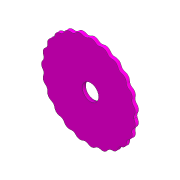
# Autodesk Inventor part: epicycloid
Saved by Autodesk Inventor 2022 (Build 260153000, 153)
## iProperties
Created: 2023-11-18
Part Number: epicycloid
Material: 一般
Document SubType Name: Modeling
Designer: JOU
Density: 1 g/cm^3
Appearance: 預設
Author: JOU
Autodesk Inventor part; units mm, degrees
ref_plane "YZ Plane" through (0, 0, 0) normal (1, 0, 0) x (0, 1, 0)
ref_plane "XZ Plane" through (0, 0, 0) normal (0, 1, 0) x (-1, 0, 0)
ref_plane "XY Plane" through (0, 0, 0) normal (0, 0, 1) x (1, 0, 0)
sketch "草圖1" plane through (0, 0, 0) normal (0, 0, 1) x (1, 0, 0)
  spline S0 degree 3 poles (138.6565, -4.115) (139.0078, -5.0402) (139.622, -6.6578) (140.7346, -8.8016) (141.6039, -10.7606) (142.2908, -12.8288) (142.7395, -15.1027) (142.8776, -17.5459) (142.6548, -20.0506) (142.0718, -22.4816) (141.1815, -24.7182) (140.0679, -26.6922) (138.8, -28.425) (137.3588, -30.0737) (135.6, -32.0105) (133.6246, -34.7946) (132.3649, -38.5247) (132.3554, -42.1634) (132.8434, -44.9603) (133.2666, -47.1894) (133.5136, -49.3089) (133.5257, -51.532) (133.2299, -53.8808) (132.5764, -56.2723) (131.5654, -58.5796) (130.2524, -60.6783) (128.7308, -62.4839) (127.0941, -63.9798) (125.3716, -65.2386) (123.4392, -66.4555) (121.0392, -68.0358) (118.3954, -70.5774) (116.5842, -74.0652) (115.9348, -77.381) (115.726, -79.9601) (115.4995, -82.13) (115.0882, -84.2405) (114.3916, -86.404) (113.3491, -88.5798) (111.9559, -90.6584) (110.2664, -92.519) (108.3804, -94.0712) (106.4106, -95.2802) (104.4306, -96.1793) (102.3977, -96.8704) (100.0593, -97.5478) (97.0906, -98.6367) (93.9043, -100.8025) (91.6334, -103.8672) (90.4103, -106.7035) (89.5885, -108.949) (88.7489, -110.9181) (87.693, -112.8302) (86.3231, -114.7076) (84.6177, -116.4688) (82.6244, -118.0035) (80.4443, -119.2217) (78.2018, -120.082) (76.0022, -120.6018) (73.8722, -120.8478) (71.6744, -120.9144) (69.029, -120.956) (65.6165, -121.4494) (62.0504, -123.1305) (59.4348, -125.6172) (57.7521, -127.8616) (56.4166, -129.6789) (55.0289, -131.3009) (53.3999, -132.8226) (51.4684, -134.2015) (49.2643, -135.3439) (46.8828, -136.1647) (44.4535, -136.6216) (42.1006, -136.7277) (39.897, -136.5414) (37.803, -136.1333) (35.5805, -135.5443) (32.7506, -134.8724) (29.059, -134.7182) (25.2982, -135.8285) (22.4771, -137.623) (20.4734, -139.2159) (18.7352, -140.5221) (16.9037, -141.6552) (14.8359, -142.614) (12.5248, -143.3247) (10.0501, -143.7098) (7.5383, -143.729) (5.1234, -143.3958) (2.9049, -142.7703) (0.9048, -141.9288) (-0.988, -140.9064) (-3.0992, -139.648) (-5.9637, -138.2247) (-9.7496, -137.4239) (-13.5121, -137.9045) (-16.3794, -138.9508) (-18.5632, -139.8737) (-20.5757, -140.5959) (-22.7016, -141.1198) (-25.0165, -141.3873) (-27.4717, -141.3277) (-29.9522, -140.9025) (-32.3231, -140.1264) (-34.4711, -139.0641) (-36.3401, -137.8045) (-37.9655, -136.4101) (-39.5172, -134.8386) (-41.3782, -132.9154) (-44.1155, -130.7638) (-47.8029, -129.3589) (-51.3772, -129.1863) (-54.132, -129.4936) (-56.3593, -129.7521) (-58.4935, -129.836) (-60.7226, -129.6717) (-63.0517, -129.1861) (-65.3888, -128.3392) (-67.6062, -127.1449) (-69.586, -125.6711) (-71.2554, -124.0184) (-72.6107, -122.2781) (-73.7347, -120.4643) (-74.8264, -118.422) (-76.2957, -115.8709) (-78.7548, -113.078) (-82.1531, -111.1423) (-85.3623, -110.3412) (-87.8678, -109.9704) (-90.0011, -109.5863) (-92.0802, -109.0105) (-94.1933, -108.1393) (-96.2872, -106.9199) (-98.2495, -105.3604) (-99.9652, -103.528) (-101.3549, -101.5309) (-102.3974, -99.4824) (-103.1361, -97.4468) (-103.6752, -95.3592) (-104.2022, -92.934) (-105.1501, -89.8407) (-107.2041, -86.5431) (-110.1376, -84.1744) (-112.8343, -82.8242) (-114.981, -81.8643) (-116.8771, -80.8802) (-118.7093, -79.6719) (-120.4808, -78.1482) (-122.1043, -76.2998) (-123.4736, -74.1873) (-124.5092, -71.9208) (-125.1834, -69.6272) (-125.5254, -67.4058) (-125.6061, -65.268) (-125.511, -63.0511) (-125.3803, -60.3469) (-125.7145, -56.8481) (-127.26, -53.2155) (-129.5824, -50.5344) (-131.6676, -48.7582) (-133.3645, -47.311) (-134.8771, -45.8009) (-136.2729, -44.0472) (-137.4984, -42.0012) (-138.4614, -39.7061) (-139.0864, -37.2668) (-139.3449, -34.8162) (-139.2628, -32.4748) (-138.9056, -30.3038) (-138.3389, -28.2455) (-137.5833, -26.0381) (-136.725, -23.1846) (-136.4072, -19.4517) (-137.3644, -15.6723) (-138.9746, -12.8244) (-140.4005, -10.7626) (-141.567, -8.9429) (-142.5579, -7.022) (-143.3536, -4.8725) (-143.8781, -2.5017) (-144.062, 0) (-143.8781, 2.5017) (-143.3536, 4.8725) (-142.5579, 7.022) (-141.567, 8.9429) (-140.4005, 10.7626) (-138.9746, 12.8244) (-137.3644, 15.6723) (-136.4072, 19.4517) (-136.725, 23.1846) (-137.5833, 26.0381) (-138.3389, 28.2455) (-138.9056, 30.3038) (-139.2628, 32.4748) (-139.3449, 34.8162) (-139.0864, 37.2668) (-138.4614, 39.7061) (-137.4984, 42.0012) (-136.2729, 44.0472) (-134.8771, 45.8009) (-133.3645, 47.311) (-131.6676, 48.7582) (-129.5824, 50.5344) (-127.26, 53.2155) (-125.7145, 56.8481) (-125.3803, 60.3469) (-125.511, 63.0511) (-125.6061, 65.268) (-125.5254, 67.4058) (-125.1834, 69.6272) (-124.5092, 71.9208) (-123.4736, 74.1873) (-122.1043, 76.2998) (-120.4808, 78.1482) (-118.7093, 79.6719) (-116.8771, 80.8802) (-114.981, 81.8643) (-112.8343, 82.8242) (-110.1376, 84.1744) (-107.2041, 86.5431) (-105.1501, 89.8407) (-104.2022, 92.934) (-103.6752, 95.3592) (-103.1361, 97.4468) (-102.3974, 99.4824) (-101.3549, 101.5309) (-99.9652, 103.528) (-98.2495, 105.3604) (-96.2872, 106.9199) (-94.1933, 108.1393) (-92.0802, 109.0105) (-90.0011, 109.5863) (-87.8678, 109.9704) (-85.3623, 110.3412) (-82.1531, 111.1423) (-78.7548, 113.078) (-76.2957, 115.8709) (-74.8264, 118.422) (-73.7347, 120.4643) (-72.6107, 122.2781) (-71.2554, 124.0184) (-69.586, 125.6711) (-67.6062, 127.1449) (-65.3888, 128.3392) (-63.0517, 129.1861) (-60.7226, 129.6717) (-58.4935, 129.836) (-56.3593, 129.7521) (-54.132, 129.4936) (-51.3772, 129.1863) (-47.8029, 129.3589) (-44.1155, 130.7638) (-41.3782, 132.9154) (-39.5172, 134.8386) (-37.9655, 136.4101) (-36.3401, 137.8045) (-34.4711, 139.0641) (-32.3231, 140.1264) (-29.9522, 140.9025) (-27.4717, 141.3277) (-25.0165, 141.3873) (-22.7016, 141.1198) (-20.5757, 140.5959) (-18.5632, 139.8737) (-16.3794, 138.9508) (-13.5121, 137.9045) (-9.7496, 137.4239) (-5.9637, 138.2247) (-3.0992, 139.648) (-0.988, 140.9064) (0.9048, 141.9288) (2.9049, 142.7703) (5.1234, 143.3958) (7.5383, 143.729) (10.0501, 143.7098) (12.5248, 143.3247) (14.8359, 142.614) (16.9037, 141.6552) (18.7352, 140.5221) (20.4734, 139.2159) (22.4771, 137.623) (25.2982, 135.8285) (29.059, 134.7182) (32.7506, 134.8724) (35.5805, 135.5443) (37.803, 136.1333) (39.897, 136.5414) (42.1006, 136.7277) (44.4535, 136.6216) (46.8828, 136.1647) (49.2643, 135.3439) (51.4684, 134.2015) (53.3999, 132.8226) (55.0289, 131.3009) (56.4166, 129.6789) (57.7521, 127.8616) (59.4348, 125.6172) (62.0504, 123.1305) (65.6165, 121.4494) (69.029, 120.956) (71.6744, 120.9144) (73.8722, 120.8478) (76.0022, 120.6018) (78.2018, 120.082) (80.4443, 119.2217) (82.6244, 118.0035) (84.6177, 116.4688) (86.3231, 114.7076) (87.693, 112.8302) (88.7489, 110.9181) (89.5885, 108.949) (90.4103, 106.7035) (91.6334, 103.8672) (93.9043, 100.8025) (97.0906, 98.6367) (100.0593, 97.5478) (102.3977, 96.8704) (104.4306, 96.1793) (106.4106, 95.2802) (108.3804, 94.0712) (110.2664, 92.519) (111.9559, 90.6584) (113.3491, 88.5798) (114.3916, 86.404) (115.0882, 84.2405) (115.4995, 82.13) (115.726, 79.9601) (115.9348, 77.381) (116.5842, 74.0652) (118.3954, 70.5774) (121.0392, 68.0358) (123.4392, 66.4555) (125.3716, 65.2386) (127.0941, 63.9798) (128.7308, 62.4839) (130.2524, 60.6783) (131.5654, 58.5796) (132.5764, 56.2723) (133.2299, 53.8808) (133.5257, 51.532) (133.5136, 49.3089) (133.2666, 47.1894) (132.8434, 44.9603) (132.3554, 42.1634) (132.3649, 38.5247) (133.6246, 34.7946) (135.6, 32.0105) (137.3588, 30.0737) (138.8, 28.425) (140.0679, 26.6922) (141.1815, 24.7182) (142.0718, 22.4816) (142.6548, 20.0506) (142.8776, 17.5459) (142.7396, 15.1027) (142.2906, 12.8289) (141.6048, 10.7602) (140.731, 8.8031) (139.6386, 6.6506) (138.4143, 3.7836) (137.7137, -0.0182) (138.3422, -2.7494) (138.6565, -4.115) knots 0 0 0 0 0.296573 0.51855 0.723917 0.939024 1.170933 1.417164 1.670651 1.922572 2.164461 2.390458 2.600664 2.80741 3.047114 3.385708 3.824889 4.202567 4.464806 4.676207 4.883237 5.104017 5.341497 5.59119 5.845157 6.09447 6.331281 6.551327 6.758018 6.970406 7.236439 7.619525 8.057124 8.39018 8.627222 8.83359 9.044347 9.271092 9.513567 9.765743 10.019093 10.264826 10.496009 10.71045 10.915801 11.139569 11.441039 11.861668 12.274181 12.565982 12.786279 12.99171 13.207495 13.440125 13.686838 13.940445 14.192096 14.433387 14.658636 14.868312 15.075502 15.318003 15.66218 16.102555 16.474742 16.733332 16.943833 17.151233 17.372751 17.610891 17.86095 18.1149 18.363816 18.599949 18.819267 19.025653 19.239117 19.50909 19.897478 20.333116 20.660693 20.895207 21.101261 21.312588 21.540081 21.78313 22.035543 22.288739 22.533961 22.764414 22.978202 23.183586 23.40926 23.715746 24.140019 24.548099 24.835259 25.053985 25.259525 25.475999 25.709343 25.956526 26.210236 26.4616 26.702282 26.926782 27.135952 27.343655 27.58909 27.938879 28.380055 28.746687 29.001773 29.211457 29.419257 29.641518 29.880308 30.130717 30.384633 30.633138 30.868585 31.08718 31.293297 31.50793 31.781987 32.175548 32.608859 32.931028 33.163144 33.368945 33.580862 33.809099 34.052711 34.305344 34.55837 34.803068 35.032786 35.245935 35.451403 35.679102 35.990716 36.418328 36.821758 37.104411 37.321672 37.527363 37.744536 37.978588 38.226226 38.480022 38.731084 38.971146 39.194897 39.403584 39.611872 39.860382 40.215796 40.657374 41.018408 41.270134 41.479081 41.687312 41.910317 42.149748 42.400492 42.654356 42.902435 43.137188 43.355068 43.560953 43.77685 44.055135 44.453716 44.884348 45.201192 45.431037 45.636643 45.849169 46.078148 46.322309 46.575147 46.827985 47.072146 47.301125 47.51365 47.719256 47.949102 48.265946 48.696577 49.095159 49.373444 49.589341 49.795226 50.013105 50.247859 50.495938 50.749802 51.000545 51.239977 51.462982 51.671212 51.880159 52.131886 52.49292 52.934498 53.289911 53.538422 53.746709 53.955396 54.179148 54.41921 54.670272 54.924068 55.171706 55.405758 55.62293 55.828622 56.045883 56.328536 56.731965 57.159578 57.471191 57.698891 57.904359 58.117508 58.347225 58.591924 58.844949 59.097583 59.341195 59.569432 59.781349 59.98715 60.219266 60.541434 60.974746 61.368306 61.642364 61.856996 62.063113 62.281708 62.517156 62.76566 63.019576 63.269985 63.508776 63.731036 63.938837 64.148521 64.403607 64.770239 65.211415 65.561204 65.806639 66.014342 66.223511 66.448011 66.688693 66.940058 67.193768 67.440951 67.674295 67.890769 68.096309 68.315035 68.602194 69.010275 69.434548 69.741034 69.966708 70.172092 70.385879 70.616332 70.861555 71.114751 71.367164 71.610213 71.837705 72.049033 72.255087 72.489601 72.817177 73.252816 73.641203 73.911176 74.12464 74.331027 74.550344 74.786477 75.035393 75.289344 75.539403 75.777543 75.999061 76.206461 76.416962 76.675552 77.047738 77.488114 77.832291 78.074792 78.281981 78.491658 78.716906 78.958197 79.209848 79.463455 79.710169 79.942799 80.158584 80.364015 80.584312 80.876113 81.288625 81.709254 82.010725 82.234493 82.439843 82.654284 82.885468 83.131201 83.384551 83.636726 83.879201 84.105947 84.316704 84.523071 84.760114 85.09317 85.530769 85.913855 86.179888 86.392276 86.598967 86.819013 87.055824 87.305136 87.559104 87.808797 88.046277 88.267057 88.474087 88.685488 88.947727 89.325405 89.764586 90.10318 90.342884 90.54963 90.759835 90.985833 91.227722 91.479643 91.73313 91.97936 92.21127 92.426377 92.631744 92.85372 93.150294 93.566996 93.983698 93.983698 93.983698 93.983698
  point P0 (0, 0)
  point P1 (140.7389, -8.8609)
  point P2 (141.5606, -10.743)
  point P3 (142.2311, -12.7869)
  point P4 (142.6787, -15.0624)
  point P5 (142.8174, -17.5208)
  point P6 (142.5929, -20.0457)
  point P7 (142.0053, -22.4955)
  point P8 (141.1112, -24.743)
  point P9 (140.0033, -26.7128)
  point P10 (138.7696, -28.4148)
  point P11 (137.4268, -29.9868)
  point P12 (135.8513, -31.7933)
  point P13 (133.9454, -34.5919)
  point P14 (132.5532, -38.7572)
  point P15 (132.4841, -42.5334)
  point P16 (132.8796, -45.1258)
  point P17 (133.2442, -47.2081)
  point P18 (133.4714, -49.2659)
  point P19 (133.479, -51.4737)
  point P20 (133.1813, -53.8298)
  point P21 (132.5231, -56.2384)
  point P22 (131.5039, -58.5646)
  point P23 (130.1815, -60.6781)
  point P24 (128.6564, -62.4897)
  point P25 (127.0352, -63.9776)
  point P26 (125.3742, -65.2077)
  point P27 (123.5938, -66.3657)
  point P28 (121.4038, -67.8761)
  point P29 (118.6823, -70.5722)
  point P30 (116.65, -74.4477)
  point P31 (115.946, -77.703)
  point P32 (115.7079, -80.0614)
  point P33 (115.4712, -82.1115)
  point P34 (115.0592, -84.1784)
  point P35 (114.3616, -86.3358)
  point P36 (113.3135, -88.5224)
  point P37 (111.9095, -90.6171)
  point P38 (110.2063, -92.4927)
  point P39 (108.3091, -94.0544)
  point P40 (106.3398, -95.2654)
  point P41 (104.3901, -96.1582)
  point P42 (102.4517, -96.8362)
  point P43 (100.3139, -97.4971)
  point P44 (97.5061, -98.5949)
  point P45 (94.0492, -100.9911)
  point P46 (91.5579, -104.279)
  point P47 (90.3452, -106.9331)
  point P48 (89.5529, -108.9887)
  point P49 (88.7318, -110.8718)
  point P50 (87.6833, -112.7577)
  point P51 (86.3107, -114.6359)
  point P52 (84.5943, -116.4082)
  point P53 (82.5849, -117.9554)
  point P54 (80.388, -119.1829)
  point P55 (78.1354, -120.0476)
  point P56 (75.944, -120.5688)
  point P57 (73.8623, -120.819)
  point P58 (71.7922, -120.9062)
  point P59 (69.3688, -120.9936)
  point P60 (65.9723, -121.5501)
  point P61 (61.9932, -123.4368)
  point P62 (59.2544, -125.957)
  point P63 (57.6596, -127.9925)
  point P64 (56.3897, -129.6713)
  point P65 (55.0323, -131.2394)
  point P66 (53.4107, -132.7485)
  point P67 (51.4719, -134.1315)
  point P68 (49.2519, -135.2822)
  point P69 (46.8509, -136.1096)
  point P70 (44.4047, -136.5697)
  point P71 (42.0458, -136.6773)
  point P72 (39.86, -136.4974)
  point P73 (37.8317, -136.1159)
  point P74 (35.7603, -135.6004)
  point P75 (33.1208, -135.0334)
  point P76 (29.2383, -134.9271)
  point P77 (25.0542, -136.1402)
  point P78 (22.2558, -137.8429)
  point P79 (20.392, -139.2662)
  point P80 (18.7316, -140.4864)
  point P81 (16.93, -141.5911)
  point P82 (14.865, -142.5456)
  point P83 (12.5418, -143.2596)
  point P84 (10.0477, -143.6478)
  point P85 (7.5158, -143.6671)
  point P86 (5.0865, -143.3321)
  point P87 (2.8679, -142.7088)
  point P88 (0.8946, -141.8863)
  point P89 (-0.9213, -140.9268)
  point P90 (-2.8805, -139.8068)
  point P91 (-5.6533, -138.5009)
  point P92 (-9.8113, -137.6574)
  point P93 (-13.8649, -138.1278)
  point P94 (-16.5831, -139.054)
  point P95 (-18.6117, -139.8716)
  point P96 (-20.5517, -140.5508)
  point P97 (-22.6549, -141.063)
  point P98 (-24.9731, -141.3293)
  point P99 (-27.4442, -141.2692)
  point P100 (-29.9449, -140.8406)
  point P101 (-32.3338, -140.0585)
  point P102 (-34.4914, -138.9921)
  point P103 (-36.355, -137.7403)
  point P104 (-37.9491, -136.386)
  point P105 (-39.4264, -134.926)
  point P106 (-41.169, -133.1977)
  point P107 (-43.9583, -131.0869)
  point P108 (-48.0831, -129.5217)
  point P109 (-51.7416, -129.2832)
  point P110 (-54.2822, -129.5125)
  point P111 (-56.3681, -129.7262)
  point P112 (-58.4449, -129.7962)
  point P113 (-60.6612, -129.6289)
  point P114 (-62.9987, -129.1407)
  point P115 (-65.353, -128.2876)
  point P116 (-67.5885, -127.0836)
  point P117 (-69.5819, -125.5997)
  point P118 (-71.256, -123.9441)
  point P119 (-72.6031, -122.2226)
  point P120 (-73.7009, -120.4781)
  point P121 (-74.7419, -118.6011)
  point P122 (-76.1606, -116.2564)
  point P123 (-78.8016, -113.3385)
  point P124 (-82.5544, -111.1721)
  point P125 (-85.6637, -110.3287)
  point P126 (-87.9529, -109.9449)
  point P127 (-89.9745, -109.5595)
  point P128 (-92.0146, -108.986)
  point P129 (-94.1237, -108.1137)
  point P130 (-96.2287, -106.8874)
  point P131 (-98.2065, -105.3157)
  point P132 (-99.9359, -103.4687)
  point P133 (-101.3338, -101.4603)
  point P134 (-102.3776, -99.4139)
  point P135 (-103.1117, -97.4129)
  point P136 (-103.6443, -95.4284)
  point P137 (-104.1691, -93.2127)
  point P138 (-105.1438, -90.2529)
  point P139 (-107.4316, -86.6403)
  point P140 (-110.539, -84.0675)
  point P141 (-113.0387, -82.7479)
  point P142 (-115.0073, -81.8288)
  point P143 (-116.8258, -80.8676)
  point P144 (-118.6356, -79.6673)
  point P145 (-120.4091, -78.1399)
  point P146 (-122.0433, -76.2793)
  point P147 (-123.4238, -74.1496)
  point P148 (-124.4671, -71.8661)
  point P149 (-125.1448, -69.5631)
  point P150 (-125.4887, -67.3522)
  point P151 (-125.5781, -65.2672)
  point P152 (-125.515, -63.1853)
  point P153 (-125.4467, -60.7011)
  point P154 (-125.8478, -57.1697)
  point P155 (-127.5784, -53.1072)
  point P156 (-129.8944, -50.3376)
  point P157 (-131.7761, -48.6654)
  point P158 (-133.3481, -47.289)
  point P159 (-134.8139, -45.81)
  point P160 (-136.1997, -44.0628)
  point P161 (-137.4294, -42.0084)
  point P162 (-138.3996, -39.6963)
  point P163 (-139.0297, -37.2371)
  point P164 (-139.2899, -34.77)
  point P165 (-139.2091, -32.4238)
  point P166 (-138.8607, -30.2731)
  point P167 (-138.3284, -28.2842)
  point P168 (-137.6618, -26.2307)
  point P169 (-136.9178, -23.5492)
  point P170 (-136.6314, -19.5737)
  point P171 (-137.661, -15.3922)
  point P172 (-139.1634, -12.6027)
  point P173 (-140.4349, -10.6879)
  point P174 (-141.5273, -8.9461)
  point P175 (-142.4947, -7.0538)
  point P176 (-143.2874, -4.9056)
  point P177 (-143.8146, -2.5216)
  point P178 (-144, 0)
  point P179 (-143.8146, 2.5216)
  point P180 (-143.2874, 4.9056)
  point P181 (-142.4947, 7.0538)
  point P182 (-141.5273, 8.9461)
  point P183 (-140.4349, 10.6879)
  point P184 (-139.1634, 12.6027)
  point P185 (-137.661, 15.3922)
  point P186 (-136.6314, 19.5737)
  point P187 (-136.9178, 23.5492)
  point P188 (-137.6618, 26.2307)
  point P189 (-138.3284, 28.2842)
  point P190 (-138.8607, 30.2731)
  point P191 (-139.2091, 32.4238)
  point P192 (-139.2899, 34.77)
  point P193 (-139.0297, 37.2371)
  point P194 (-138.3996, 39.6963)
  point P195 (-137.4294, 42.0084)
  point P196 (-136.1997, 44.0628)
  point P197 (-134.8139, 45.81)
  point P198 (-133.3481, 47.289)
  point P199 (-131.7761, 48.6654)
  constraints: 360 other
extrude "擠出1" add sketch "草圖1" along normal blind 10
sketch "草圖2" plane through (0, 0, 10) normal (0, 0, 1) x (1, 0, 0)
  circle A0 centre (6, 0) radius 25
  point P0 (0, 0)
  dimension "d2" = 6
  dimension "d3" = 50
  constraints: 1 centre point
  measures "d2" distance of point (0, 0) A0.centre
  measures "d3" diameter of A0
extrude "擠出2" cut sketch "草圖2" against normal blind 10
